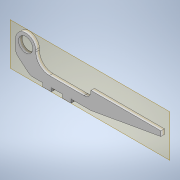
# Autodesk Inventor part: cuerpo_chapa
Saved by Autodesk Inventor 2021 (Build 250183000, 183)
## iProperties
Created: 2026-06-23
Part Number: cuerpo_chapa
Material: Generic
Document SubType Name: Sheet Metal
Designer: nelso
Density: 1 g/cm^3
Sheet Metal Rule: Default_mm
Appearance: Default
Author: nelso
Autodesk Inventor part; units mm, degrees
ref_plane "YZ Plane" through (0, 0, 0) normal (1, 0, 0) x (0, 1, 0)
ref_plane "XZ Plane" through (0, 0, 0) normal (0, 1, 0) x (-1, 0, 0)
sketch "Sketch1" plane through (0, 0, 0) normal (0, 0, 1) x (1, 0, 0)
  line L0 (57.892, -6.3043) -> (120, -6.3043)
  line L1 (120, -6.3043) -> (120, -10.6498)
  line L2 (120, -10.6498) -> (57.892, -21.6998)
  line L3 (4.088, -21.6998) -> (15.288, -21.6998)
  line L4 (15.288, -21.6998) -> (15.288, -24.8998)
  line L5 (15.288, -24.8998) -> (22.788, -24.8998)
  line L6 (22.788, -24.8998) -> (22.788, -21.6998)
  line L7 (32.788, -21.6998) -> (32.788, -24.8998)
  line L8 (40.288, -24.8998) -> (40.288, -21.6998)
  circle A0 centre (0, 0) radius 6.35
  circle A1 centre (0, 0) radius 9
  line L9 (57.892, -6.3043) -> (120, -6.3043)
  line L10 (120, -6.3043) -> (120, -10.6498)
  line L11 (57.892, -21.6998) -> (120, -10.6498)
  line L12 (57.892, -21.6998) -> (40.288, -21.6998)
  line L13 (40.288, -24.8998) -> (40.288, -21.6998)
  line L14 (40.288, -24.8998) -> (32.788, -24.8998)
  line L15 (32.788, -24.8998) -> (32.788, -21.6998)
  line L16 (32.788, -21.6998) -> (22.788, -21.6998)
  line L17 (22.788, -24.8998) -> (22.788, -21.6998)
  line L18 (15.288, -24.8998) -> (22.788, -24.8998)
  line L19 (15.288, -24.8998) -> (15.288, -21.6998)
  line L20 (15.288, -21.6998) -> (4.088, -21.6998)
  line L21 (57.892, -6.3043) -> (57.892, -13.3043)
  line L22 (57.892, -13.3043) -> (8.9781, -13.3043)
  line L23 (8.9781, 0.6275) -> (8.9781, -13.3043)
  line L24 (-9, 0) -> (-9, -10.6498)
  line L25 (-9, -10.6498) -> (4.088, -21.6998)
  dimension "d1" = 11.2
  dimension "d2" = 7.5
  dimension "d3" = 10
  dimension "d4" = 7.5
  dimension "d8" = 12.7
  dimension "d15" = 21.6998
  dimension "d20" = 7
  dimension "d21" = 57.892
  dimension "d22" = 120
  dimension "d24" = 18
  dimension "d25" = 17.604
  dimension "d27" = 4.088
  measures "d1" distance of L3.start L3.end
  measures "d2" distance of L4.end L5.end
  measures "d3" distance of L6.end L7.start
  measures "d4" distance of L7.end L8.start
  measures "d8" diameter of A0
  measures "d15" distance from line of L3 A0.centre
  measures "d20" distance of L0.start L21.end
  measures "d21" distance from line of L21 A0.centre
  measures "d22" distance from line of A0.centre L1
  measures "d24" diameter of A1
  measures "d25" distance of L2.end L8.end
  measures "d27" horizontal distance of L3.start A0.centre
extrude "Plate1" add sketch "Sketch1" along normal mid plane 3.2 contours L0 L1 L2 L12 L8 L14 L7 L16 L6 L5 L4 L3 L25 L24 A1 L23 L22 L21 | A1 L23 picked at (-8.0333, -0.7023)
fillet "Corner Round1" radius 12 1 edges at (8.9781, -13.3043, 0)
fillet "Corner Round2" radius 6 2 edges at (-9, -10.6498, 0) (4.088, -21.6998, 0)
fillet "Corner Round3" radius 6 1 edges at (57.892, -13.3043, 0)
equation "\"d4\" = d2"
equation "\"d0\" = Thickness"
equation "\"BendRadius\" = Thickness"
equation "\"BendReliefWidth\" = Thickness"
equation "\"BendReliefDepth\" = 0.5 * Thickness"
equation "\"CornerReliefSize\" = 4 * Thickness"
equation "\"MinimumRemnant\" = 2 * Thickness"
equation "\"TransitionRadius\" = BendRadius"
equation "\"JacobiRadiusSize\" = BendRadius"
equation "\"GapSize\" = Thickness"
equation "\"Thickness\" = 3.2"
body "Solid1"
